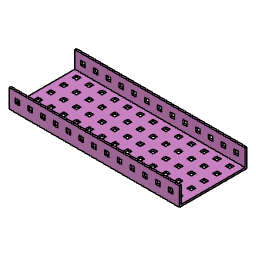
lead screw assembly v3 (Autodesk Fusion 360 archive; units mm, degrees)
design "base"
Autodesk Fusion 360 part; units mm, degrees
sketch "Sketch1" plane through (0, 0, 0) normal (0, 0, 1) x (1, 0, 0)
  line L0 (0, 0) -> (200, 0)
  line L1 (200, 0) -> (200, 79)
  line L2 (200, 79) -> (0, 79)
  line L3 (0, 79) -> (0, 0)
  dimension "d1" = 200
  dimension "d2" = 79
  constraint horizontal L0
  constraint vertical L1
  constraint horizontal L2
  constraint vertical L3
  constraint coincident L0.start L3.end
  measures "d1" distance of L0.start L0.end
  measures "d2" distance of L0.start L2.end
extrude "Extrude1" add sketch "Sketch1" along normal blind 2
sketch "Sketch2" plane through (0, 0, 2) normal (0, 0, 1) x (-1, 0, 0)
  line L0 (0, -79) -> (0, 0)
  line L1 (0, 0) -> (-200, 0)
  line L2 (-200, 0) -> (-200, -79)
  line L3 (-200, -79) -> (0, -79)
  line L4 (0, -79) -> (-200, -79)
  line L5 (-200, -79) -> (-200, -77)
  line L6 (-200, -77) -> (0, -77)
  line L7 (0, -77) -> (0, -79)
  line L8 (0, -39.5) -> (-200, -39.5) construction
  line L9 (0, 0) -> (-200, 0)
  line L10 (-200, -2) -> (0, -2)
  dimension "d5" = 2
  constraint horizontal L4
  constraint vertical L5
  constraint horizontal L6
  constraint vertical L7
  constraint coincident L0.start L3.end
  constraint midpoint L0 L8.start
  constraint midpoint L2 L8.end
  constraint symmetric L0.start L8 L0.end
  constraint symmetric L2.end L8 L1.end
  constraint symmetric L5.end L8 L10.start
  constraint symmetric L6.end L8 L10.end
  measures "d5" distance of L0.start L6.end
extrude "Extrude2" add sketch "Sketch2" along normal blind 20 contours L0 L2 L3 L4 L5 L6 L7 | L0 L1 L2 L9 L10
sketch "Sketch3" plane through (0, 0, 0) normal (0, 0, -1) x (1, 0, 0)
  line L0 (0, 0) -> (0, -79)
  line L1 (0, -79) -> (200, -79)
  line L2 (200, -79) -> (200, 0)
  line L3 (200, 0) -> (0, 0)
  line L4 (7, -7) -> (12, -7)
  line L5 (12, -7) -> (12, -12)
  line L6 (12, -12) -> (7, -12)
  line L7 (7, -12) -> (7, -7)
  dimension "d8" = 5
  dimension "d9" = 5
  dimension "d10" = 7
  dimension "d11" = 7
  constraint horizontal L4
  constraint vertical L5
  constraint horizontal L6
  constraint vertical L7
  measures "d8" distance of L4.start L4.end
  measures "d9" distance of L4.start L6.end
  measures "d10" distance of L3 L4
  measures "d11" distance of L0 L7
extrude "Extrude3" cut sketch "Sketch3" against normal blind 2 contours L4 L5 L6 L7
pattern_linear "R-Pattern1" count 13 spacing 15 along (1, 0, 0) count 5 spacing 15 along (0, 1, 0) of "Extrude3"
ref_plane "WorkPlane1" through (100, 39.5, 11) normal (0, 1, 0) x (-1, 0, 0)
sketch "Sketch4" plane through (0, 0, 0) normal (0, -1, 0) x (1, 0, 0)
  line L0 (0, 0) -> (200, 0)
  line L1 (200, 0) -> (200, 22)
  line L2 (200, 22) -> (0, 22)
  line L3 (0, 22) -> (0, 0)
  line L4 (0, 2) -> (200, 2) construction
  line L5 (7, 14.5) -> (12, 14.5)
  line L6 (12, 14.5) -> (12, 9.5)
  line L7 (12, 9.5) -> (7, 9.5)
  line L8 (7, 9.5) -> (7, 14.5)
  dimension "d18" = 2
  dimension "d19" = 5
  dimension "d20" = 5
  dimension "d21" = 7
  dimension "d22" = 7.5
  constraint coincident L3 L4.start
  constraint coincident L1 L4.end
  constraint perpendicular L1 L4
  constraint horizontal L5
  constraint vertical L6
  constraint horizontal L7
  constraint vertical L8
  measures "d18" distance of L0 L4
  measures "d19" distance of L5.start L5.end
  measures "d20" distance of L5.start L7.end
  measures "d21" distance of L3 L8
  measures "d22" distance of L2 L5
extrude "Extrude4" cut sketch "Sketch4" against normal blind 2 contours L5 L6 L7 L8
pattern_linear "R-Pattern2" count 13 spacing 15 along (1, 0, 0) of "Extrude4"
mirror "Mirror1" about plane through (100, 39.5, 11) normal (0, 1, 0) of "Extrude4", "R-Pattern2"
equation "d2 = 75 mm + 2 * 2 mm"

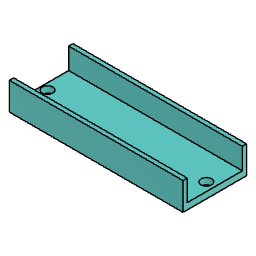
design "sled"
Autodesk Fusion 360 part; units mm, degrees
sketch "Sketch1" plane through (0, 0, 0) normal (0, 0, 1) x (1, 0, 0)
  line L0 (0, 0) -> (82, 0)
  line L1 (82, 0) -> (82, 30)
  line L2 (82, 30) -> (0, 30)
  line L3 (0, 30) -> (0, 0)
  dimension "d1" = 82
  dimension "d2" = 30
  constraint horizontal L0
  constraint vertical L1
  constraint horizontal L2
  constraint vertical L3
  constraint coincident L0.start L3.end
  measures "d1" distance of L0.start L0.end
  measures "d2" distance of L0.start L2.end
extrude "Extrude1" add sketch "Sketch1" along normal blind 3
sketch "Sketch2" plane through (0, 0, 3) normal (0, 0, 1) x (-1, 0, 0)
  line L0 (0, -30) -> (0, 0)
  line L1 (0, 0) -> (-82, 0)
  line L2 (-82, 0) -> (-82, -30)
  line L3 (-82, -30) -> (0, -30)
  line L4 (0, -30) -> (-82, -30)
  line L5 (-82, -30) -> (-82, -28)
  line L6 (-82, -28) -> (0, -28)
  line L7 (0, -28) -> (0, -30)
  line L8 (0, 0) -> (-82, 0)
  line L9 (-82, 0) -> (-82, -2)
  line L10 (-82, -2) -> (0, -2)
  line L11 (0, -2) -> (0, 0)
  dimension "d5" = 2
  dimension "d6" = 2
  dimension "d15" = 82
  dimension "d16" = 82
  dimension "d17" = 82
  constraint horizontal L4
  constraint vertical L5
  constraint horizontal L6
  constraint vertical L7
  constraint coincident L0.start L3.end
  constraint horizontal L8
  constraint vertical L9
  constraint horizontal L10
  constraint vertical L11
  constraint coincident L0.end L1.start
  measures "d5" distance of L0.start L6.end
  measures "d6" distance of L0.end L10.end
  measures "d15" distance of L0.start L2.end
  measures "d16" distance of L0.start L2.end
  measures "d17" distance of L9.end L10.end
extrude "Extrude2" add sketch "Sketch2" along normal blind 10 contours L0 L2 L3 L4 L5 L6 L7 | L0 L1 L2 L8 L9 L10 L11
sketch "Sketch3" plane through (0, 0, 3) normal (0, 0, 1) x (-1, 0, 0)
  line L0 (-82, -28) -> (0, -28)
  line L1 (0, -28) -> (0, -2)
  line L2 (0, -2) -> (-82, -2)
  line L3 (-82, -2) -> (-82, -28)
  circle A0 centre (-3, -15) radius 2.5
  dimension "d9" = 5
  dimension "d10" = 3
  dimension "d11" = 13
  dimension "d12" = 26
  measures "d9" diameter of A0
  measures "d10" distance of L1 A0.centre
  measures "d11" distance of L2 A0.centre
  measures "d12" distance of L0.end L1.end
extrude "Extrude3" cut sketch "Sketch3" against normal blind 3 contours A0
pattern_linear "R-Pattern1" count 2 spacing 75 along (1, 0, 0) of "Extrude3"
equation "d11 = d12 / 2"
equation "d15 = d16"
equation "d17 = d16"

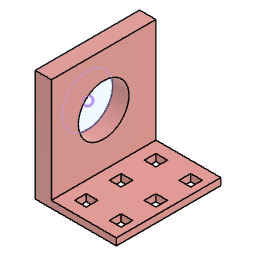
design "bearingbracketballs and back"
Autodesk Fusion 360 part; units mm, degrees
sketch "Sketch1" plane through (0, 0, 0) normal (0, 0, 1) x (1, 0, 0)
  line L0 (0, 0) -> (35, 0)
  line L1 (35, 0) -> (35, 45)
  line L2 (35, 45) -> (0, 45)
  line L3 (0, 45) -> (0, 0)
  dimension "d1" = 35
  dimension "d2" = 45
  constraint horizontal L0
  constraint vertical L1
  constraint horizontal L2
  constraint vertical L3
  constraint coincident L0.start L3.end
  measures "d1" distance of L0.start L0.end
  measures "d2" distance of L0.start L2.end
extrude "Extrude1" add sketch "Sketch1" along normal blind 3
sketch "Sketch2" plane through (0, 0, 3) normal (0, 0, 1) x (-1, 0, 0)
  line L0 (0, -45) -> (0, 0)
  line L1 (0, 0) -> (-35, 0)
  line L2 (-35, 0) -> (-35, -45)
  line L3 (-35, -45) -> (0, -45)
  line L4 (0, -45) -> (-7, -45)
  line L5 (-7, -45) -> (-7, 0)
  line L6 (-7, 0) -> (0, 0)
  line L7 (0, 0) -> (0, -45)
  dimension "d5" = 7
  constraint horizontal L4
  constraint vertical L5
  constraint horizontal L6
  constraint vertical L7
  constraint coincident L0.start L3.end
  measures "d5" distance of L0.start L4.end
extrude "Extrude2" add sketch "Sketch2" along normal blind 45 contours L0 L1 L3 L4 L5 L6 L7
sketch "Sketch3" plane through (0, 0, 3) normal (0, 0, 1) x (-1, 0, 0)
  line L0 (-7, -45) -> (-7, 0)
  line L1 (-7, 0) -> (-35, 0)
  line L2 (-35, 0) -> (-35, -45)
  line L3 (-35, -45) -> (-7, -45)
  line L4 (-12, -40) -> (-17, -40)
  line L5 (-17, -40) -> (-17, -35)
  line L6 (-17, -35) -> (-12, -35)
  line L7 (-12, -35) -> (-12, -40)
  dimension "d8" = 5
  dimension "d9" = 5
  dimension "d10" = 5
  dimension "d11" = 5
  constraint horizontal L4
  constraint vertical L5
  constraint horizontal L6
  constraint vertical L7
  measures "d8" distance of L4.start L4.end
  measures "d9" distance of L4.start L6.end
  measures "d10" distance of L3 L4
  measures "d11" distance of L0 L7
extrude "Extrude3" cut sketch "Sketch3" against normal blind 3 contours L4 L5 L6 L7
pattern_linear "R-Pattern1" count 3 spacing 15 along (1, 0, 0) count 3 spacing 15 along (0, -1, 0) of "Extrude3"
sketch "Sketch4" plane through (7, 0, 0) normal (1, 0, 0) x (0, 1, 0)
  line L0 (0, 3) -> (45, 3)
  line L1 (45, 3) -> (45, 48)
  line L2 (45, 48) -> (0, 48)
  line L3 (0, 48) -> (0, 3)
  line L4 (22.5, 48) -> (22.5, 3) construction
  line L5 (0, 25.5) -> (45, 25.5) construction
  circle A0 centre (22.5, 25.5) radius 10.9
  dimension "d18" = 21.8
  constraint midpoint L2 L4.start
  constraint midpoint L0 L4.end
  constraint midpoint L3 L5.start
  constraint midpoint L1 L5.end
  constraint midpoint L5 A0.centre
  measures "d18" diameter of A0
extrude "Extrude4" cut sketch "Sketch4" against normal blind 7 contours A0
sketch "Sketch5" plane through (0, 0, 0) normal (-1, 0, 0) x (0, -1, 0)
  line L0 (-45, 0) -> (0, 0)
  line L1 (0, 0) -> (0, 48)
  line L2 (0, 48) -> (-45, 48)
  line L3 (-45, 48) -> (-45, 0)
  circle A0 centre (-22.5, 25.5) radius 10.9

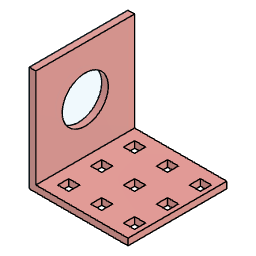
design "handle bracket balls and back"
Autodesk Fusion 360 part; units mm, degrees
sketch "Sketch1" plane through (0, 0, 0) normal (0, 0, 1) x (1, 0, 0)
  line L0 (0, 0) -> (45, 0)
  line L1 (45, 0) -> (45, 45)
  line L2 (45, 45) -> (0, 45)
  line L3 (0, 45) -> (0, 0)
  dimension "d1" = 45
  dimension "d2" = 45
  constraint horizontal L0
  constraint vertical L1
  constraint horizontal L2
  constraint vertical L3
  constraint coincident L0.start L3.end
  measures "d1" distance of L0.start L0.end
  measures "d2" distance of L0.start L2.end
extrude "Extrude1" add sketch "Sketch1" along normal blind 3
sketch "Sketch2" plane through (0, 0, 3) normal (0, 0, 1) x (-1, 0, 0)
  line L0 (0, -45) -> (0, 0)
  line L1 (0, 0) -> (-45, 0)
  line L2 (-45, 0) -> (-45, -45)
  line L3 (-45, -45) -> (0, -45)
  line L4 (0, -45) -> (-3, -45)
  line L5 (-3, -45) -> (-3, 0)
  line L6 (-3, 0) -> (0, 0)
  line L7 (0, 0) -> (0, -45)
  dimension "d5" = 3
  constraint horizontal L4
  constraint vertical L5
  constraint horizontal L6
  constraint vertical L7
  constraint coincident L0.start L3.end
  measures "d5" distance of L0.start L4.end
extrude "Extrude2" add sketch "Sketch2" along normal blind 45 contours L0 L1 L3 L4 L5 L6 L7
sketch "Sketch3" plane through (0, 0, 3) normal (0, 0, 1) x (-1, 0, 0)
  line L0 (-3, -45) -> (-3, 0)
  line L1 (-3, 0) -> (-45, 0)
  line L2 (-45, 0) -> (-45, -45)
  line L3 (-45, -45) -> (-3, -45)
  line L4 (-8, -40) -> (-13, -40)
  line L5 (-13, -40) -> (-13, -35)
  line L6 (-13, -35) -> (-8, -35)
  line L7 (-8, -35) -> (-8, -40)
  dimension "d8" = 5
  dimension "d9" = 5
  dimension "d10" = 5
  dimension "d11" = 5
  constraint horizontal L4
  constraint vertical L5
  constraint horizontal L6
  constraint vertical L7
  measures "d8" distance of L4.start L4.end
  measures "d9" distance of L4.start L6.end
  measures "d10" distance of L3 L4
  measures "d11" distance of L0 L7
extrude "Extrude3" cut sketch "Sketch3" against normal blind 3 contours L4 L5 L6 L7
pattern_linear "R-Pattern1" count 3 spacing 15 along (1, 0, 0) count 3 spacing 15 along (0, -1, 0) of "Extrude3"
sketch "Sketch4" plane through (3, 0, 0) normal (1, 0, 0) x (0, 1, 0)
  line L0 (0, 3) -> (45, 3)
  line L1 (45, 3) -> (45, 48)
  line L2 (45, 48) -> (0, 48)
  line L3 (0, 48) -> (0, 3)
  line L4 (22.5, 48) -> (22.5, 3) construction
  line L5 (0, 25.5) -> (45, 25.5) construction
  circle A0 centre (22.5, 25.5) radius 10.5
  dimension "d18" = 21
  constraint midpoint L2 L4.start
  constraint midpoint L0 L4.end
  constraint midpoint L3 L5.start
  constraint midpoint L1 L5.end
  constraint midpoint L5 A0.centre
  measures "d18" diameter of A0
extrude "Extrude4" cut sketch "Sketch4" against normal blind 3 contours A0
sketch "Sketch5" plane through (0, 0, 0) normal (-1, 0, 0) x (0, -1, 0)
  circle A0 centre (-22.5, 25.5) radius 10.5
  line L0 (-45, 0) -> (0, 0)
  line L1 (0, 0) -> (0, 48)
  line L2 (0, 48) -> (-45, 48)
  line L3 (-45, 48) -> (-45, 0)
